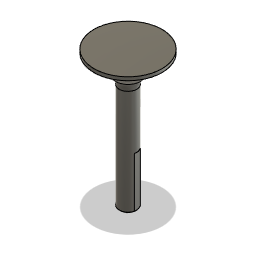
Parametric Object Mount Shaft for Openscan Mini v2 (Autodesk Fusion 360 design; units mm, degrees)
Autodesk Fusion 360 part; units mm, degrees
sketch "Shaft Thickness" plane through (0, 0, 0) normal (0, 1, 0) x (1, 0, 0)
  circle A0 centre (0, 0) radius 5.175
  dimension "Shaft_Thickness" = 10.35
  constraint coincident A0.centre origin
  measures "Shaft_Thickness" diameter of A0
ref_plane "WorkPlane1" through (0, 15, 0) normal (0, 1, 0) x (1, 0, 0)
sketch "Top mount Circle where objects sit" plane through (0, 15, 0) normal (0, 1, 0) x (1, 0, 0)
  circle A0 centre (0, 0) radius 20
  dimension "Top_Mount_Diameter" = 40
  constraint coincident A0.centre origin
  measures "Top_Mount_Diameter" diameter of A0
loft "Loft1" add profiles "Top mount Circle where objects sit", "Shaft Thickness" section 1 section 2
extrude "Shaft Length" add 1 faces at (0.1289, 0, 1.7202) along direction (0, -1, 0) blind 65
sketch "Sketch3" plane through (0, -65, 0) normal (0, -1, 0) x (-1, 0, 0)
  circle A0 centre (0, 0) radius 5.175
  line L0 (-1.7948, 1.8114) -> (-2.3287, -1.039)
  arc A1 (-2.3287, -1.039) -> (-1.7948, 1.8114) centre (0, 0) ccw
  line L1 (-5.0216, -1.2505) -> (-4.1018, 3.1553)
  arc A2 (-5.0216, -1.2505) -> (-4.1018, 3.1553) centre (0, 0) ccw
  dimension "d8" = 5.1
  dimension "d9" = 2.9
  constraint coincident A0.centre A1.centre
  measures "d8" diameter of A1
  measures "d9" distance of L0.end L0.start
extrude "Cutout for Stepper Motor Shaft" cut sketch "Sketch3" against normal blind 30 contours A0 L1 | L0 A1
extrude "Thicker Object Mounting Area" add 1 faces at (4.7423, 15, 7.1112) along direction (0, -1, 0) blind 2
fillet "Fillet to Smooth Top to Shaft" radius 7 2 edges at (-16.8036, 13, -6.5175) (-4.8248, 0, 1.8714)
chamfer "Chamfer top aid insertion" distance 0.65 angle 45 3 edges at (-5.0658, -65, 1.0576) (2.0618, -65, -0.3862) (-2.5064, -65, 0.4695)
fillet "Fillet2" radius 2.15 2 edges at (-2.5064, -35, 0.4695) (2.0618, -64.35, -0.3862)
equation "Shaft_Thickness = 10.35 mm" comment "Slightly thinner than stock to stop grinding on rotor"
equation "Topmount_to_shaft_distance = 15 mm" comment "The length of slope from top mount to shaft start, default 15mm"
equation "Top_Mount_Diameter = 40 mm" comment "The diameter of the disc/circle on top of shaft. Make smaller for long mounts for tiny things"
equation "Shaft_Length = 80 mm - Topmount_to_shaft_distance" comment "Takes into account the length of Topmount to Shaft distance"
equation "Cutout_StepperMotor = -30 mm" comment "Most stepper motor shafts are around 25mm so you have 5mm to spare"
equation "Lip_Thickness_TopCircle = -2 mm"
equation "Fillet_Top_to_Shaft = 7 mm"
equation "Chamfer_Stepper_Aid = 0.65 mm"
equation "Fillet_inside_shaft = 2.15 mm" comment "Used to ensure no supports needed if printed upside down!"
